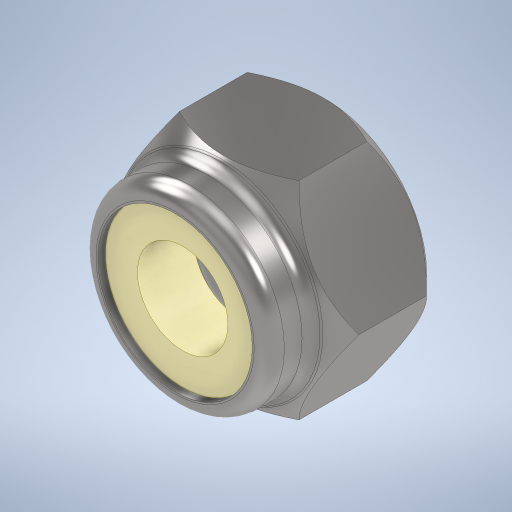
# Autodesk Inventor part: M3 LOCKNUT
Saved by Autodesk Inventor 2024 (Build 280153000, 153)
## iProperties
Created: 2024-09-05
Part Number: M3 LOCKNUT
Material: Stainless Steel
Document SubType Name: Modeling
Designer: Ishaan
Density: 8 g/cm^3
Appearance: Semi-Polished
Author: Ishaan
Autodesk Inventor part; units mm, degrees
ref_plane "YZ Plane" through (0, 0, 0) normal (1, 0, 0) x (0, 1, 0)
ref_plane "XZ Plane" through (0, 0, 0) normal (0, 1, 0) x (-1, 0, 0)
ref_plane "XY Plane" through (0, 0, 0) normal (0, 0, 1) x (1, 0, 0)
sketch "Sketch1" plane through (0, 0, 0) normal (0, 0, 1) x (1, 0, 0)
  circle A0 centre (0, 0) radius 3.175426
  line L0 (-1.587713, 2.75) -> (1.587713, 2.75)
  line L1 (1.587713, 2.75) -> (3.175426, 0)
  line L2 (3.175426, 0) -> (1.587713, -2.75)
  line L3 (1.587713, -2.75) -> (-1.587713, -2.75)
  line L4 (-1.587713, -2.75) -> (-3.175426, 0)
  line L5 (-3.175426, 0) -> (-1.587713, 2.75)
  point P0 (-3.175426, 0)
  point P1 (-3.175426, 0)
  point P2 (-1.587713, 2.75)
  point P3 (-1.587713, 2.75)
  point P4 (-1.587713, -2.75)
  point P5 (-1.587713, -2.75)
  point P6 (3.175426, 0)
  point P7 (3.175426, 0)
  point P8 (1.587713, -2.75)
  dimension "d0" = 5.5
  constraints: 12 end point, 2 coincident, 1 horizontal, 16 other
  measures "d0" distance between parallel lines of L3 L0
extrude "Extrusion1" add sketch "Sketch1" along normal blind 2.8
chamfer "Chamfer1" distance 0.5 angle 45 2 edges at (-3.1754, 0, 0) (-3.1754, 0, 2.8)
extrude "Extrusion2" cut sketch "Sketch1" along normal through all contours L1 A0 | A0 L2 | L0 A0 | A0 L3 | L5 A0 | A0 L4
sketch "Sketch2" plane through (0, 0, 2.8) normal (0, 0, 1) x (1, 0, 0)
  circle A0 centre (0, 0) radius 2.675426
  circle A1 centre (0, 0) radius 2.5
  dimension "d9" = 5
  constraints: 1 centre point, 1 coincident
  measures "d9" diameter of A1
extrude "Extrusion3" add sketch "Sketch2" along normal blind 1.2 contours A1
fillet "Fillet1" radius 0.4 3 edges at (-2.5, 0, 2.8) (-2.6754, 0, 2.8) (-2.5, 0, 4)
sketch "Sketch3" plane through (0, 0, 4) normal (0, 0, 1) x (1, 0, 0)
  circle A0 centre (0, 0) radius 2.05
  dimension "d13" = 4.1
  constraints: 1 centre point, 1 coincident
  measures "d13" diameter of A0
extrude "Extrusion4" cut sketch "Sketch3" against normal blind 1.7
sketch "Sketch4" plane through (0, 0, 2.3) normal (0, 0, 1) x (1, 0, 0)
  circle A0 centre (0, 0) radius 2.05 projected
extrude "Extrusion5" add sketch "Sketch4" along normal blind 1.5 separate body
sketch "Sketch5" plane through (0, 0, 3.8) normal (0, 0, 1) x (1, 0, 0)
  circle A0 centre (0, 0) radius 2.05 projected
  constraints: 1 coincident
hole "Hole1" at (0, 0, 3.8) direction (0, 0, -1) diameter 2.459 end through all bodies 1 thread size "M3x0.5" class "6H" standard "ANSI Metric M Profile"
sketch "Sketch6" plane through (0, 0, 2.3) normal (0, 0, -1) x (-1, 0, 0)
  circle A0 centre (0, 0) radius 1.2295 projected
  constraints: 1 coincident
hole "Hole2" at (0, 0, 2.3) direction (0, 0, 1) diameter 2.4 end through all bodies 2
chamfer "Chamfer2" distance 0.2 angle 45 1 edges at (0, 1.2295, 0)
body "Solid1"
